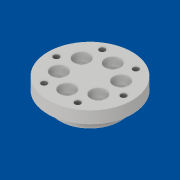
# Autodesk Inventor part: 405-output disk
Saved by Autodesk Inventor 2018 (Build 220112000, 112)
## iProperties
Created: 2020-06-21
Part Number: 405-output disk
Material: Generic
Document SubType Name: Modeling
Designer: Bunny320
Density: 1 g/cm^3
Appearance: Default
Author: Bunny320
Autodesk Inventor part; units mm, degrees
ref_plane "YZ Plane" through (0, 0, 0) normal (1, 0, 0) x (0, 1, 0)
ref_plane "XZ Plane" through (0, 0, 0) normal (0, 1, 0) x (-1, 0, 0)
ref_plane "XY Plane" through (0, 0, 0) normal (0, 0, 1) x (1, 0, 0)
sketch "Sketch1" plane through (0, 0, 0) normal (0, 1, 0) x (-1, 0, 0)
  line L0 (13.5, 4) -> (13.5, 5)
  line L1 (13.5, 5) -> (17.5, 5)
  line L2 (17.5, 5) -> (17.5, 10)
  line L3 (17.5, 10) -> (0, 10)
  line L4 (0, 10) -> (0, 0)
  line L5 (13.5, 4) -> (12.5, 4)
  line L6 (12.5, 4) -> (12.5, 0)
  line L7 (12.5, 0) -> (0, 0)
  dimension "d1" = 27
  dimension "d2" = 35
  dimension "d3" = 1
  dimension "d4" = 5
  dimension "d28" = 25
  dimension "d29" = 4
  constraints: 16 end point, 6 perpendicular, 1 horizontal, 1 vertical
  measures "d1" diameter of L0 L4
  measures "d2" diameter of L2 L4
  measures "d3" distance of L0.start L0.end
  measures "d4" distance of L1.end L2.end
  measures "d28" diameter of L6 L4
  measures "d29" distance of L5.end L6.end
revolve "Revolution1" add sketch "Sketch1" angle 360 about axis through (0, 0, 10) along (0, 0, -1)
sketch "Sketch2" plane through (0, 0, 10) normal (0, 0, 1) x (1, 0, 0)
  point P0 (0, 0)
  point P1 (0, 9.5)
  dimension "d6" = 9.5
  constraints: 1 vertical alignment
  measures "d6" distance of point (0, 0) point (0, 9.5)
hole "Hole1" at (0, 9.5, 10) direction (0, 0, -1) diameter 3.4 end through all counterbore diameter 6.5 counterbore depth 4 clearance for "Socket Head Cap Screw DIN EN ISO 4762" size "M3" standard "DIN"
pattern_circular "Circular Pattern1" count 6 over 360 about axis through (0, 0, -10) along (0, 0, -1) of "Hole1"
sketch "Sketch3" plane through (0, 0, 10) normal (0, 0, 1) x (1, 0, 0)
  point P0 (0, 0)
  point P1 (14, 0)
  dimension "d17" = 14
  constraints: 1 horizontal alignment
  measures "d17" distance of point (0, 0) point (14, 0)
hole "Hole2" at (14, 0, 10) direction (0, 0, -1) diameter 2.459 end through all thread size "M3x0.5" class "6H" standard "ISO Metric profile"
pattern_circular "Circular Pattern2" count 6 over 360 about axis through (0, 0, -10) along (0, 0, 1) of "Hole2"
body "Solid1"
